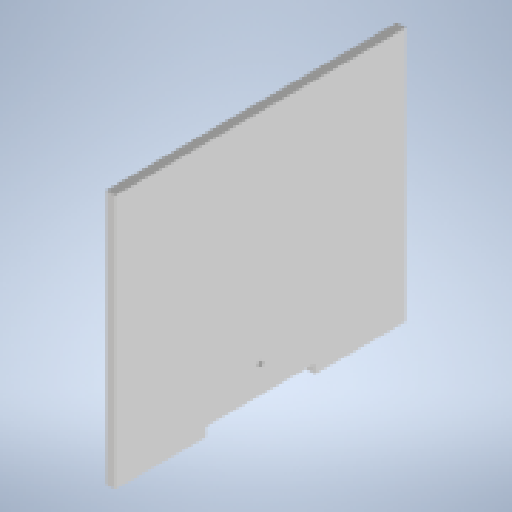
# Autodesk Inventor part: TOP_1
Saved by Autodesk Inventor 2025.3 (Build 293356030, 356C)
## iProperties
Created: 2026-06-30
Part Number: TOP_1
Material: Generic
Document SubType Name: Modeling
Designer: user
Density: 1 g/cm^3
Appearance: Default
Mass: 131.064 g
Surface Area: 474.149 cm^2
Volume: 110.323 cm^3
Author: user
Autodesk Inventor part; units mm, degrees
ref_plane "YZ Plane" through (0, 0, 0) normal (1, 0, 0) x (0, 1, 0)
ref_plane "XZ Plane" through (0, 0, 0) normal (0, 1, 0) x (-1, 0, 0)
ref_plane "XY Plane" through (0, 0, 0) normal (0, 0, 1) x (1, 0, 0)
sketch "Sketch1" plane through (0, 0, 0) normal (1, 0, 0) x (0, 1, 0)
  line L0 (0, 0) -> (140, 0)
  line L1 (140, 0) -> (140, -160)
  line L2 (140, -160) -> (0, -160)
  line L3 (0, -160) -> (0, 0)
  line L4 (0, -50) -> (5, -50)
  line L5 (5, -50) -> (5, -110)
  line L6 (5, -110) -> (0, -110)
  line L7 (0, -110) -> (0, -50)
  point P0 (0, -110)
  dimension "d0" = 140
  dimension "d1" = 160
  dimension "d2" = 5
  dimension "d3" = 60
  dimension "d4" = 50
  constraints: 16 end point, 4 parallel, 2 horizontal, 2 perpendicular, 1 point on line
  measures "d0" distance of L1.end L2.end
  measures "d1" distance of L0.end L1.end
  measures "d2" distance of L5.end L6.end
  measures "d3" distance of L4.end L5.end
  measures "d4" distance between parallel lines of L0 L4
extrude "Extrusion1" add sketch "Sketch1" along normal blind 5 contours L0 L1 L2 L3 L6 L5 L4
sketch "Sketch2" plane through (5, 0, 0) normal (1, 0, 0) x (0, 0, -1)
  line L0 (0, 0) -> (50, 0) projected
  line L1 (50, 0) -> (50, 5) projected
  point P0 (80, 20)
  dimension "d14" = 20
  dimension "d15" = 30
  measures "d14" distance from line of L0 point (80, 20)
  measures "d15" distance from line of point (80, 20) L1
hole "Hole1" at (5, 20, -80) direction (-1, 0, 0) diameter 3 end through all
sketch "Sketch12" plane through (5, 0, 0) normal (1, 0, 0) x (0, 0, -1)
  circle A0 centre (95.2983, 42.3183) radius 1.5 projected
  circle A1 centre (92.9456, 121.5257) radius 1.5 projected
  circle A2 centre (70.9676, 122.7958) radius 1.5 projected
  circle A3 centre (66.5863, 42.8118) radius 1.5 projected
  point P0 (0, 0)
extrude "Extrusion5" cut sketch "Sketch12" against normal through all
body "Solid1"
